Autodesk Inventor part; units mm, degrees
(part 2 of 2)
  arc A186 (143.0168, 108.2996) -> (148.9586, 106.0969) centre (168.8384, 168.8384) ccw
  arc A187 (149.6716, 82.58) -> (149.6716, 89.42) centre (146.2516, 86) ccw
  arc A188 (142.8316, 89.42) -> (142.8316, 82.58) centre (146.2516, 86) ccw
  arc A189 (129.9116, 82.58) -> (129.9116, 89.42) centre (126.4916, 86) ccw
  arc A190 (162.6162, 88.8364) -> (163.108, 82.58) centre (166.574, 86) ccw
  arc A191 (162.6162, 88.8364) -> (162.6167, 91.1656) centre (160.9905, 90.0014) ccw
  arc A192 (162.2055, 96.1467) -> (162.6167, 91.1656) centre (166.576, 94) ccw
  arc A193 (162.2055, 96.1467) -> (161.7567, 96.8671) centre (161.7567, 96.3671) ccw
  arc A194 (161.208, 75.1329) -> (163.108, 77.0329) centre (161.208, 77.0329) ccw
  arc A195 (149.6716, 77.0329) -> (151.5716, 75.1329) centre (151.5716, 77.0329) ccw
  line L125 (151.5716, 96.8671) -> (161.7567, 96.8671)
  line L126 (163.108, 82.58) -> (163.108, 77.0329)
  line L127 (161.208, 75.1329) -> (151.5716, 75.1329)
  line L128 (149.6716, 77.0329) -> (149.6716, 82.58)
  arc A196 (140.9316, 75.1329) -> (142.8316, 77.0329) centre (140.9316, 77.0329) ccw
  arc A197 (138.1595, 75.3626) -> (139.0651, 75.1329) centre (139.0651, 77.0329) ccw
  arc A198 (129.9116, 80.9656) -> (130.906, 79.2953) centre (131.8116, 80.9656) ccw
  arc A199 (130.906, 92.7047) -> (129.9116, 91.0344) centre (131.8116, 91.0344) ccw
  arc A200 (142.8316, 94.9671) -> (140.9316, 96.8671) centre (140.9316, 94.9671) ccw
  arc A201 (139.0651, 96.8671) -> (138.1595, 96.6374) centre (139.0651, 94.9671) ccw
  line L129 (130.906, 92.7047) -> (138.1595, 96.6374)
  line L130 (139.0651, 96.8671) -> (140.9316, 96.8671)
  line L131 (142.8316, 94.9671) -> (142.8316, 89.42)
  line L132 (142.8316, 82.58) -> (142.8316, 77.0329)
  line L133 (138.1595, 75.3626) -> (130.906, 79.2953)
  line L134 (129.9116, 80.9656) -> (129.9116, 82.58)
  line L135 (129.9116, 89.42) -> (129.9116, 91.0344)
  line L136 (139.0651, 75.1329) -> (140.9316, 75.1329)
  arc A202 (131.2701, 73.3555) -> (131.3324, 75.1447) centre (130.8558, 74.2656) ccw
  arc A203 (122.2131, 80.089) -> (118.7118, 78.848) centre (121.0215, 77.8913) ccw
  arc A204 (112.9272, 64.8827) -> (113.8511, 63.5) centre (113.8511, 64.5) ccw
  arc A205 (115.4267, 63.5) -> (116.072, 63.7361) centre (115.4267, 64.5) ccw
  arc A206 (131.2701, 73.3555) -> (116.072, 63.7361) centre (158.5315, 13.4685) ccw
  line L137 (115.4267, 63.5) -> (113.8511, 63.5)
  line L138 (112.9272, 64.8827) -> (118.7118, 78.848)
  line L139 (122.2131, 80.089) -> (131.3324, 75.1447)
  arc A207 (122.1239, 65.314) -> (122.7047, 63.5) centre (122.7047, 64.5) ccw
  arc A208 (148.9522, 65.9007) -> (150.6725, 68.8) centre (148.0207, 68.4135) ccw
  arc A209 (142.036, 63.5) -> (143.0168, 63.7004) centre (142.036, 66) ccw
  arc A210 (136.55, 72.3159) -> (134.8209, 72.401) centre (135.5967, 70.5576) ccw
  arc A211 (138.308, 71.3627) -> (139.7379, 71) centre (139.7379, 74) ccw
  line L140 (139.7379, 71) -> (146.5, 71)
  line L141 (146.5, 71) -> (146.5, 68.8)
  line L142 (146.5, 68.8) -> (150.6725, 68.8)
  line L143 (148.9522, 65.9007) -> (143.0168, 63.7004)
  line L144 (142.036, 63.5) -> (122.7047, 63.5)
  line L145 (138.308, 71.3627) -> (136.55, 72.3159)
  arc A212 (134.8209, 72.401) -> (122.1239, 65.314) centre (160.3459, 11.7536) ccw
  arc A213 (89.42, 29.1684) -> (82.58, 29.1684) centre (86, 25.7484) ccw
  arc A214 (82.58, 22.3284) -> (89.42, 22.3284) centre (86, 25.7484) ccw
  arc A215 (82.58, 42.0884) -> (89.42, 42.0884) centre (86, 45.5084) ccw
  arc A216 (75.1329, 10.792) -> (77.0329, 8.892) centre (77.0329, 10.792) ccw
  arc A217 (96.8671, 20.4284) -> (94.9671, 22.3284) centre (94.9671, 20.4284) ccw
  arc A218 (77.0329, 22.3284) -> (75.1329, 20.4284) centre (77.0329, 20.4284) ccw
  line L146 (77.0329, 22.3284) -> (82.58, 22.3284)
  line L147 (89.42, 22.3284) -> (94.9671, 22.3284)
  line L148 (75.1329, 20.4284) -> (75.1329, 10.792)
  line L149 (77.0329, 8.892) -> (82.58, 8.892)
  arc A219 (96.1467, 9.7945) -> (96.8671, 10.2433) centre (96.3671, 10.2433) ccw
  arc A220 (96.1467, 9.7945) -> (91.1656, 9.3833) centre (94, 5.424) ccw
  arc A221 (88.8364, 9.3838) -> (91.1656, 9.3833) centre (90.0014, 11.0095) ccw
  arc A222 (88.8364, 9.3838) -> (82.58, 8.892) centre (86, 5.426) ccw
  line L150 (96.8671, 10.2433) -> (96.8671, 20.4284)
  arc A223 (94.9671, 29.1684) -> (96.8671, 31.0684) centre (94.9671, 31.0684) ccw
  arc A224 (96.8671, 32.9349) -> (96.6374, 33.8405) centre (94.9671, 32.9349) ccw
  arc A225 (75.1329, 31.0684) -> (77.0329, 29.1684) centre (77.0329, 31.0684) ccw
  arc A226 (75.3626, 33.8405) -> (75.1329, 32.9349) centre (77.0329, 32.9349) ccw
  arc A227 (80.9656, 42.0884) -> (79.2953, 41.094) centre (80.9656, 40.1884) ccw
  arc A228 (92.7047, 41.094) -> (91.0344, 42.0884) centre (91.0344, 40.1884) ccw
  line L151 (96.8671, 32.9349) -> (96.8671, 31.0684)
  line L152 (94.9671, 29.1684) -> (89.42, 29.1684)
  line L153 (96.6374, 33.8405) -> (92.7047, 41.094)
  line L154 (91.0344, 42.0884) -> (89.42, 42.0884)
  line L155 (82.58, 42.0884) -> (80.9656, 42.0884)
  line L156 (79.2953, 41.094) -> (75.3626, 33.8405)
  line L157 (75.1329, 32.9349) -> (75.1329, 31.0684)
  line L158 (77.0329, 29.1684) -> (82.58, 29.1684)
  arc A229 (119.0041, 59.6222) -> (118.6767, 60.5) centre (118.6767, 60) ccw
  arc A230 (114, 60.5) -> (111.5, 58) centre (114, 58) ccw
  arc A231 (111.5, 53.3233) -> (112.3778, 52.9958) centre (112, 53.3233) ccw
  line L159 (114, 60.5) -> (118.6767, 60.5)
  line L160 (111.5, 58) -> (111.5, 53.3233)
  arc A232 (119.0041, 59.6222) -> (112.3778, 52.9958) centre (162.1005, 9.8995) ccw
  arc A233 (123.9045, 60.5) -> (122.6628, 60.0679) centre (123.9045, 58.5) ccw
  arc A234 (111.9321, 49.3372) -> (111.5, 48.0955) centre (113.5, 48.0955) ccw
  arc A235 (133.455, 58.6568) -> (132.9173, 60.5) centre (132.9173, 59.5) ccw
  arc A236 (111.5, 39.0827) -> (113.3432, 38.545) centre (112.5, 39.0827) ccw
  line L161 (111.5, 39.0827) -> (111.5, 48.0955)
  arc A237 (122.6628, 60.0679) -> (111.9321, 49.3372) centre (163.5147, 8.4853) ccw
  arc A238 (133.455, 58.6568) -> (113.3432, 38.545) centre (168.8384, 3.1616) ccw
  line L162 (132.9173, 60.5) -> (123.9045, 60.5)
  arc A239 (93.152, 53.2882) -> (91.911, 49.7869) centre (94.1087, 50.9785) ccw
  arc A240 (108.5, 58.1489) -> (107.1173, 59.0728) centre (107.5, 58.1489) ccw
  arc A241 (108.2639, 55.928) -> (108.5, 56.5733) centre (107.5, 56.5733) ccw
  arc A242 (96.8553, 40.6676) -> (98.6445, 40.7299) centre (97.7344, 41.1442) ccw
  arc A243 (108.2639, 55.928) -> (98.6445, 40.7299) centre (158.5315, 13.4685) ccw
  line L163 (108.5, 56.5733) -> (108.5, 58.1489)
  line L164 (107.1173, 59.0728) -> (93.152, 53.2882)
  line L165 (91.911, 49.7869) -> (96.8553, 40.6676)
  arc A244 (101, 32.2621) -> (100.6373, 33.692) centre (98, 32.2621) ccw
  arc A245 (99.599, 37.1791) -> (99.6841, 35.45) centre (101.4423, 36.4033) ccw
  arc A246 (108.2996, 28.9832) -> (108.5, 29.964) centre (106, 29.964) ccw
  arc A247 (103.2, 21.3275) -> (106.0968, 23.0414) centre (103.5865, 23.9793) ccw
  arc A248 (108.5, 49.2953) -> (106.686, 49.8761) centre (107.5, 49.2953) ccw
  arc A249 (106.686, 49.8761) -> (99.599, 37.1791) centre (160.2464, 11.6541) ccw
  line L166 (108.5, 49.2953) -> (108.5, 29.964)
  line L167 (100.6373, 33.692) -> (99.6841, 35.45)
  arc A250 (108.2996, 28.9832) -> (106.0968, 23.0414) centre (168.8384, 3.1616) ccw
  line L168 (103.2, 21.3275) -> (103.2, 25.5)
  line L169 (103.2, 25.5) -> (101, 25.5)
  line L170 (101, 25.5) -> (101, 32.2621)
  arc A251 (65.9031, 23.0414) -> (68.8, 21.3275) centre (68.4135, 23.9793) ccw
  arc A252 (63.5, 29.964) -> (63.7004, 28.9832) centre (66, 29.964) ccw
  arc A253 (71.3627, 33.692) -> (71, 32.2621) centre (74, 32.2621) ccw
  arc A254 (72.3159, 35.45) -> (72.401, 37.1791) centre (70.5576, 36.4033) ccw
  arc A255 (65.314, 49.8761) -> (63.5, 49.2953) centre (64.5, 49.2953) ccw
  arc A256 (65.9031, 23.0414) -> (63.7004, 28.9832) centre (3.1615, 3.1616) ccw
  arc A257 (72.401, 37.1791) -> (65.314, 49.8761) centre (11.7536, 11.6541) ccw
  line L171 (68.8, 21.3275) -> (68.8, 25.5)
  line L172 (68.8, 25.5) -> (71, 25.5)
  line L173 (71, 25.5) -> (71, 32.2621)
  line L174 (71.3627, 33.692) -> (72.3159, 35.45)
  line L175 (63.5, 29.964) -> (63.5, 49.2953)
  arc A258 (80.089, 49.7869) -> (78.848, 53.2882) centre (77.8913, 50.9785) ccw
  arc A259 (64.8827, 59.0728) -> (63.5, 58.1489) centre (64.5, 58.1489) ccw
  arc A260 (63.5, 56.5733) -> (63.7361, 55.928) centre (64.5, 56.5733) ccw
  arc A261 (73.3555, 40.7299) -> (75.1447, 40.6676) centre (74.2656, 41.1442) ccw
  line L176 (75.1447, 40.6676) -> (80.089, 49.7869)
  line L177 (78.848, 53.2882) -> (64.8827, 59.0728)
  line L178 (63.5, 58.1489) -> (63.5, 56.5733)
  arc A262 (73.3555, 40.7299) -> (63.7361, 55.928) centre (13.4685, 13.4685) ccw
  arc A263 (151.5716, 96.8671) -> (149.6716, 94.9671) centre (151.5716, 94.9671) ccw
  line L179 (149.6716, 94.9671) -> (149.6716, 89.42)
  arc A264 (91.911, 122.2131) -> (93.152, 118.7118) centre (94.1087, 121.0215) ccw
  line L180 (93.152, 118.7118) -> (107.1173, 112.9272)
  arc A265 (75.8533, 162.2055) -> (80.8344, 162.6167) centre (78, 166.576) ccw
  arc A266 (75.8533, 162.2055) -> (75.1329, 161.7567) centre (75.6329, 161.7567) ccw
  line L181 (75.1329, 161.7567) -> (75.1329, 151.5716)
  arc A267 (75.1329, 139.0651) -> (75.3626, 138.1595) centre (77.0329, 139.0651) ccw
  line L182 (75.1329, 139.0651) -> (75.1329, 140.9316)
  line L183 (75.3626, 138.1595) -> (79.2953, 130.906)
  arc A268 (63.6264, 105.803) -> (61.8724, 104.5705) centre (63.7201, 103.8052) ccw
  arc A269 (67.4295, 110.1276) -> (66.197, 108.3735) centre (68.1948, 108.2799) ccw
  arc A270 (63.6264, 105.803) -> (66.197, 108.3735) centre (63.5, 108.5) ccw
  arc A271 (61.8724, 67.4295) -> (63.6264, 66.197) centre (63.7201, 68.1948) ccw
  arc A272 (66.197, 63.6265) -> (67.4295, 61.8724) centre (68.1948, 63.7201) ccw
  arc A273 (66.197, 63.6265) -> (63.6264, 66.197) centre (63.5, 63.5) ccw
  line L184 (67.4295, 61.8724) -> (82.0705, 55.8078)
  line L185 (61.8724, 67.4295) -> (55.8078, 82.0705)
  line L186 (55.8078, 89.9295) -> (61.8724, 104.5705)
  line L187 (67.4295, 110.1276) -> (82.0705, 116.1922)
  arc A274 (82.0705, 55.8078) -> (84.1823, 56.1767) centre (82.8359, 57.6556) ccw
  arc A275 (87.8177, 56.1767) -> (89.9295, 55.8078) centre (89.1641, 57.6556) ccw
  arc A276 (87.8177, 56.1767) -> (84.1823, 56.1767) centre (86, 54.1802) ccw
  line L188 (89.9295, 55.8078) -> (104.5705, 61.8724)
  arc A277 (31.0684, 96.8671) -> (29.1684, 94.9671) centre (31.0684, 94.9671) ccw
  line L189 (31.0684, 96.8671) -> (32.9349, 96.8671)
  line L190 (29.1684, 89.42) -> (29.1684, 94.9671)
  circle A278 centre (54.1802, 86) radius 1.6
  circle A279 centre (63.5, 108.5) radius 1.6
  circle A280 centre (86, 117.8198) radius 1.6
  circle A281 centre (108.5, 108.5) radius 1.6
  circle A282 centre (117.8198, 86) radius 1.6
  circle A283 centre (108.5, 63.5) radius 1.6
  circle A284 centre (63.5, 63.5) radius 1.6
  circle A285 centre (86, 54.1802) radius 1.6
  arc A286 (56.1767, 84.1823) -> (56.1767, 87.8177) centre (54.1802, 86) ccw
  arc A287 (55.8078, 89.9295) -> (56.1767, 87.8177) centre (57.6556, 89.1641) ccw
  arc A288 (56.1767, 84.1823) -> (55.8078, 82.0705) centre (57.6556, 82.8359) ccw
  arc A289 (63.6264, 105.803) -> (66.197, 108.3735) centre (63.5, 108.5) ccw
  arc A290 (63.6264, 105.803) -> (61.8724, 104.5705) centre (63.7201, 103.8052) ccw
  arc A291 (67.4295, 110.1276) -> (66.197, 108.3735) centre (68.1948, 108.2799) ccw
  arc A292 (84.1823, 115.8233) -> (87.8177, 115.8233) centre (86, 117.8198) ccw
  arc A293 (89.9295, 116.1922) -> (87.8177, 115.8233) centre (89.1641, 114.3444) ccw
  arc A294 (84.1823, 115.8233) -> (82.0705, 116.1922) centre (82.8359, 114.3444) ccw
  arc A295 (105.803, 108.3735) -> (108.3735, 105.803) centre (108.5, 108.5) ccw
  arc A296 (110.1276, 104.5705) -> (108.3735, 105.803) centre (108.2799, 103.8052) ccw
  arc A297 (105.803, 108.3735) -> (104.5705, 110.1276) centre (103.8052, 108.2799) ccw
  arc A298 (115.8233, 87.8177) -> (115.8233, 84.1823) centre (117.8198, 86) ccw
  arc A299 (116.1922, 82.0705) -> (115.8233, 84.1823) centre (114.3444, 82.8359) ccw
  arc A300 (115.8233, 87.8177) -> (116.1922, 89.9295) centre (114.3444, 89.1641) ccw
  arc A301 (66.197, 63.6265) -> (63.6264, 66.197) centre (63.5, 63.5) ccw
  arc A302 (61.8724, 67.4295) -> (63.6264, 66.197) centre (63.7201, 68.1948) ccw
  arc A303 (66.197, 63.6265) -> (67.4295, 61.8724) centre (68.1948, 63.7201) ccw
  arc A304 (87.8177, 56.1767) -> (84.1823, 56.1767) centre (86, 54.1802) ccw
  arc A305 (82.0705, 55.8078) -> (84.1823, 56.1767) centre (82.8359, 57.6556) ccw
  arc A306 (87.8177, 56.1767) -> (89.9295, 55.8078) centre (89.1641, 57.6556) ccw
  arc A307 (108.3735, 66.197) -> (105.803, 63.6265) centre (108.5, 63.5) ccw
  arc A308 (104.5705, 61.8724) -> (105.803, 63.6265) centre (103.8052, 63.7201) ccw
  arc A309 (108.3735, 66.197) -> (110.1276, 67.4295) centre (108.2799, 68.1948) ccw
  line L191 (55.8078, 82.0705) -> (61.8724, 67.4295)
  line L192 (67.4295, 61.8724) -> (82.0705, 55.8078)
  line L193 (89.9295, 55.8078) -> (104.5705, 61.8724)
  line L194 (110.1276, 67.4295) -> (116.1922, 82.0705)
  line L195 (116.1922, 89.9295) -> (110.1276, 104.5705)
  line L196 (104.5705, 110.1276) -> (89.9295, 116.1922)
  line L197 (82.0705, 116.1922) -> (67.4295, 110.1276)
  line L198 (61.8724, 104.5705) -> (55.8078, 89.9295)
  line L199 (0, 99.484) -> (0, 101)
  arc A310 (0, 99.484) -> (0.217, 98.5779) centre (2, 99.484) ccw
  line L200 (0, 101) -> (6.5, 101)
  line L201 (6.5, 101) -> (6.5, 103.2)
  line L202 (6.5, 103.2) -> (0, 103.2)
  line L203 (0, 103.2) -> (0, 106.2)
  line L204 (71, 172) -> (71, 165.5)
  line L205 (71, 165.5) -> (68.8, 165.5)
  line L206 (68.8, 165.5) -> (68.8, 172)
  line L207 (68.8, 172) -> (65.8, 172)
  arc A311 (0, 106.2) -> (65.8, 172) centre (0, 172) ccw
  line L208 (101, 172) -> (101, 165.5)
  line L209 (101, 165.5) -> (103.2, 165.5)
  line L210 (103.2, 165.5) -> (103.2, 172)
  line L211 (103.2, 172) -> (106.2, 172)
  line L212 (172, 101) -> (165.5, 101)
  line L213 (165.5, 101) -> (165.5, 103.2)
  line L214 (165.5, 103.2) -> (172, 103.2)
  line L215 (172, 103.2) -> (172, 106.2)
  arc A312 (106.2, 172) -> (172, 106.2) centre (172, 172) ccw
  line L216 (0, 71) -> (6.5, 71)
  line L217 (6.5, 71) -> (6.5, 68.8)
  line L218 (6.5, 68.8) -> (0, 68.8)
  line L219 (0, 68.8) -> (0, 65.8)
  line L220 (71, 0) -> (71, 6.5)
  line L221 (71, 6.5) -> (68.8, 6.5)
  line L222 (68.8, 6.5) -> (68.8, 0)
  line L223 (68.8, 0) -> (65.8, 0)
  arc A313 (65.8, 0) -> (0, 65.8) centre (0, 0) ccw
  line L224 (101, 0) -> (101, 6.5)
  line L225 (101, 6.5) -> (103.2, 6.5)
  line L226 (103.2, 6.5) -> (103.2, 0)
  line L227 (103.2, 0) -> (106.2, 0)
  line L228 (172, 71) -> (165.5, 71)
  line L229 (165.5, 71) -> (165.5, 68.8)
  line L230 (165.5, 68.8) -> (172, 68.8)
  line L231 (172, 68.8) -> (172, 65.8)
  arc A314 (172, 65.8) -> (106.2, 0) centre (172, 0) ccw
  circle A315 centre (45.5084, 86) radius 2.1
  circle A316 centre (5.472, 86) radius 1.6
  circle A317 centre (25.7484, 86) radius 1.6
  line L232 (10.792, 96.8671) -> (20.4284, 96.8671)
  arc A318 (10.792, 96.8671) -> (8.892, 94.9671) centre (10.792, 94.9671) ccw
  line L233 (8.892, 94.9671) -> (8.892, 89.42)
  line L234 (22.3284, 89.42) -> (22.3284, 94.9671)
  arc A319 (22.3284, 94.9671) -> (20.4284, 96.8671) centre (20.4284, 94.9671) ccw
  line L235 (10.2433, 75.1329) -> (20.4284, 75.1329)
  line L236 (22.3284, 82.58) -> (22.3284, 77.0329)
  arc A320 (20.4284, 75.1329) -> (22.3284, 77.0329) centre (20.4284, 77.0329) ccw
  arc A321 (9.3838, 83.1636) -> (8.892, 89.42) centre (5.426, 86) ccw
  arc A322 (22.3284, 89.42) -> (22.3284, 82.58) centre (25.7484, 86) ccw
  line L237 (32.9349, 96.8671) -> (31.0684, 96.8671)
  line L238 (29.1684, 89.42) -> (29.1684, 94.9671)
  arc A323 (31.0684, 96.8671) -> (29.1684, 94.9671) centre (31.0684, 94.9671) ccw
  arc A324 (29.1684, 82.58) -> (29.1684, 89.42) centre (25.7484, 86) ccw
  line L239 (33.8405, 96.6374) -> (41.094, 92.7047)
  arc A325 (33.8405, 96.6374) -> (32.9349, 96.8671) centre (32.9349, 94.9671) ccw
  line L240 (42.0884, 91.0344) -> (42.0884, 89.42)
  arc A326 (42.0884, 91.0344) -> (41.094, 92.7047) centre (40.1884, 91.0344) ccw
  arc A327 (42.0884, 89.42) -> (42.0884, 82.58) centre (45.5084, 86) ccw
  line L241 (32.9349, 75.1329) -> (31.0684, 75.1329)
  line L242 (29.1684, 82.58) -> (29.1684, 77.0329)
  arc A328 (29.1684, 77.0329) -> (31.0684, 75.1329) centre (31.0684, 77.0329) ccw
  line L243 (33.8405, 75.3626) -> (41.094, 79.2953)
  arc A329 (32.9349, 75.1329) -> (33.8405, 75.3626) centre (32.9349, 77.0329) ccw
  line L244 (42.0884, 80.9656) -> (42.0884, 82.58)
  arc A330 (41.094, 79.2953) -> (42.0884, 80.9656) centre (40.1884, 80.9656) ccw
  circle A331 centre (126.4916, 86) radius 2.1
  circle A332 centre (146.2516, 86) radius 1.6
  line L245 (161.7567, 96.8671) -> (151.5716, 96.8671)
  line L246 (149.6716, 89.42) -> (149.6716, 94.9671)
  arc A333 (151.5716, 96.8671) -> (149.6716, 94.9671) centre (151.5716, 94.9671) ccw
  line L247 (161.208, 75.1329) -> (151.5716, 75.1329)
  line L248 (149.6716, 82.58) -> (149.6716, 77.0329)
  arc A334 (149.6716, 77.0329) -> (151.5716, 75.1329) centre (151.5716, 77.0329) ccw
  arc A335 (149.6716, 82.58) -> (149.6716, 89.42) centre (146.2516, 86) ccw
  line L249 (139.0651, 96.8671) -> (140.9316, 96.8671)
  line L250 (142.8316, 89.42) -> (142.8316, 94.9671)
  arc A336 (142.8316, 94.9671) -> (140.9316, 96.8671) centre (140.9316, 94.9671) ccw
  arc A337 (142.8316, 89.42) -> (142.8316, 82.58) centre (146.2516, 86) ccw
  line L251 (138.1595, 96.6374) -> (130.906, 92.7047)
  arc A338 (139.0651, 96.8671) -> (138.1595, 96.6374) centre (139.0651, 94.9671) ccw
  line L252 (129.9116, 91.0344) -> (129.9116, 89.42)
  arc A339 (130.906, 92.7047) -> (129.9116, 91.0344) centre (131.8116, 91.0344) ccw
  arc A340 (129.9116, 82.58) -> (129.9116, 89.42) centre (126.4916, 86) ccw
  line L253 (139.0651, 75.1329) -> (140.9316, 75.1329)
  line L254 (142.8316, 82.58) -> (142.8316, 77.0329)
  arc A341 (140.9316, 75.1329) -> (142.8316, 77.0329) centre (140.9316, 77.0329) ccw
  line L255 (138.1595, 75.3626) -> (130.906, 79.2953)
  arc A342 (138.1595, 75.3626) -> (139.0651, 75.1329) centre (139.0651, 77.0329) ccw
  line L256 (129.9116, 80.9656) -> (129.9116, 82.58)
  arc A343 (129.9116, 80.9656) -> (130.906, 79.2953) centre (131.8116, 80.9656) ccw
  circle A344 centre (86, 126.4916) radius 2.1
  circle A345 centre (86, 146.2516) radius 1.6
  line L257 (75.1329, 161.7567) -> (75.1329, 151.5716)
  line L258 (82.58, 149.6716) -> (77.0329, 149.6716)
  arc A346 (75.1329, 151.5716) -> (77.0329, 149.6716) centre (77.0329, 151.5716) ccw
  line L259 (96.8671, 161.208) -> (96.8671, 151.5716)
  line L260 (89.42, 149.6716) -> (94.9671, 149.6716)
  arc A347 (94.9671, 149.6716) -> (96.8671, 151.5716) centre (94.9671, 151.5716) ccw
  arc A348 (89.42, 149.6716) -> (82.58, 149.6716) centre (86, 146.2516) ccw
  line L261 (75.1329, 139.0651) -> (75.1329, 140.9316)
  line L262 (82.58, 142.8316) -> (77.0329, 142.8316)
  arc A349 (77.0329, 142.8316) -> (75.1329, 140.9316) centre (77.0329, 140.9316) ccw
  arc A350 (82.58, 142.8316) -> (89.42, 142.8316) centre (86, 146.2516) ccw
  line L263 (75.3626, 138.1595) -> (79.2953, 130.906)
  arc A351 (75.1329, 139.0651) -> (75.3626, 138.1595) centre (77.0329, 139.0651) ccw
  arc A352 (96.8671, 20.4284) -> (94.9671, 22.3284) centre (94.9671, 20.4284) ccw
  line L264 (80.9656, 129.9116) -> (82.58, 129.9116)
  arc A353 (79.2953, 130.906) -> (80.9656, 129.9116) centre (80.9656, 131.8116) ccw
  arc A354 (89.42, 129.9116) -> (82.58, 129.9116) centre (86, 126.4916) ccw
  line L265 (96.8671, 139.0651) -> (96.8671, 140.9316)
  line L266 (89.42, 142.8316) -> (94.9671, 142.8316)
  arc A355 (96.8671, 140.9316) -> (94.9671, 142.8316) centre (94.9671, 140.9316) ccw
  line L267 (96.6374, 138.1595) -> (92.7047, 130.906)
  line L268 (96.8671, 32.9349) -> (96.8671, 31.0684)
  arc A356 (96.6374, 138.1595) -> (96.8671, 139.0651) centre (94.9671, 139.0651) ccw
  line L269 (91.0344, 129.9116) -> (89.42, 129.9116)
  arc A357 (91.0344, 129.9116) -> (92.7047, 130.906) centre (91.0344, 131.8116) ccw
  circle A358 centre (86, 45.5084) radius 2.1
  circle A359 centre (86, 25.7484) radius 1.6
  line L270 (96.8671, 10.2433) -> (96.8671, 20.4284)
  line L271 (89.42, 22.3284) -> (94.9671, 22.3284)
  line L272 (75.1329, 10.792) -> (75.1329, 20.4284)
  arc A360 (92.7047, 41.094) -> (91.0344, 42.0884) centre (91.0344, 40.1884) ccw
  line L273 (82.58, 22.3284) -> (77.0329, 22.3284)
  line L274 (82.58, 29.1684) -> (77.0329, 29.1684)
  arc A361 (77.0329, 22.3284) -> (75.1329, 20.4284) centre (77.0329, 20.4284) ccw
  arc A362 (82.58, 22.3284) -> (89.42, 22.3284) centre (86, 25.7484) ccw
  line L275 (80.9656, 42.0884) -> (82.58, 42.0884)
  line L276 (89.42, 29.1684) -> (94.9671, 29.1684)
  arc A363 (94.9671, 29.1684) -> (96.8671, 31.0684) centre (94.9671, 31.0684) ccw
  arc A364 (89.42, 29.1684) -> (82.58, 29.1684) centre (86, 25.7484) ccw
  line L277 (96.6374, 33.8405) -> (92.7047, 41.094)
  arc A365 (96.8671, 32.9349) -> (96.6374, 33.8405) centre (94.9671, 32.9349) ccw
  line L278 (91.0344, 42.0884) -> (89.42, 42.0884)
  arc A366 (82.58, 42.0884) -> (89.42, 42.0884) centre (86, 45.5084) ccw
  line L279 (75.1329, 32.9349) -> (75.1329, 31.0684)
  arc A367 (75.1329, 31.0684) -> (77.0329, 29.1684) centre (77.0329, 31.0684) ccw
  arc A368 (80.9656, 42.0884) -> (79.2953, 41.094) centre (80.9656, 40.1884) ccw
  line L280 (75.3626, 33.8405) -> (79.2953, 41.094)
  arc A369 (75.3626, 33.8405) -> (75.1329, 32.9349) centre (77.0329, 32.9349) ccw
  line L281 (2.052, 94.4881) -> (2.052, 89.42)
  arc A370 (2.052, 89.42) -> (1.5587, 83.1656) centre (5.518, 86) ccw
  line L282 (0.217, 98.5779) -> (1.835, 95.3941)
  arc A371 (2.052, 94.4881) -> (1.835, 95.3941) centre (0.052, 94.4881) ccw
  arc A372 (0.217, 73.4221) -> (0, 72.516) centre (2, 72.516) ccw
  line L283 (0.217, 73.4221) -> (0.8629, 74.6931)
  line L284 (0, 71) -> (0, 72.516)
  circle A373 centre (5.47, 78) radius 1.6
  arc A374 (9.7945, 75.8533) -> (9.3832, 80.8344) centre (5.424, 78) ccw
  arc A375 (9.7945, 75.8533) -> (10.2433, 75.1329) centre (10.2433, 75.6329) ccw
  arc A376 (9.3838, 83.1636) -> (9.3832, 80.8344) centre (11.0095, 81.9986) ccw
  arc A377 (1.5581, 80.8364) -> (0.9538, 76.2982) centre (5.516, 78) ccw
  arc A378 (1.5581, 80.8364) -> (1.5587, 83.1656) centre (-0.0675, 82.0014) ccw
  arc A379 (0.8629, 74.6931) -> (0.9538, 76.2982) centre (-0.9201, 75.5992) ccw
  line L285 (172, 72.516) -> (172, 71)
  arc A380 (172, 72.516) -> (171.783, 73.4221) centre (170, 72.516) ccw
  circle A381 centre (166.528, 86) radius 1.6
  arc A382 (161.208, 75.1329) -> (163.108, 77.0329) centre (161.208, 77.0329) ccw
  line L286 (163.108, 77.0329) -> (163.108, 82.58)
  arc A383 (162.6162, 88.8364) -> (163.108, 82.58) centre (166.574, 86) ccw
  line L287 (169.948, 77.5119) -> (169.948, 82.58)
  arc A384 (169.948, 82.58) -> (170.4413, 88.8344) centre (166.482, 86) ccw
  line L288 (171.783, 73.4221) -> (170.165, 76.6059)
  arc A385 (169.948, 77.5119) -> (170.165, 76.6059) centre (171.948, 77.5119) ccw
  arc A386 (171.783, 98.5779) -> (172, 99.484) centre (170, 99.484) ccw
  line L289 (171.783, 98.5779) -> (171.1371, 97.3069)
  line L290 (172, 101) -> (172, 99.484)
  circle A387 centre (166.53, 94) radius 1.6
  arc A388 (162.2055, 96.1467) -> (162.6167, 91.1656) centre (166.576, 94) ccw
  arc A389 (162.2055, 96.1467) -> (161.7567, 96.8671) centre (161.7567, 96.3671) ccw
  arc A390 (162.6162, 88.8364) -> (162.6167, 91.1656) centre (160.9905, 90.0014) ccw
  arc A391 (170.4419, 91.1636) -> (171.0462, 95.7018) centre (166.484, 94) ccw
  arc A392 (170.4419, 91.1636) -> (170.4413, 88.8344) centre (172.0675, 89.9986) ccw
  arc A393 (171.1371, 97.3069) -> (171.0462, 95.7018) centre (172.92, 96.4008) ccw
  line L291 (72.516, 0) -> (71, 0)
  arc A394 (72.516, 0) -> (73.4221, 0.217) centre (72.516, 2) ccw
  circle A395 centre (86, 5.472) radius 1.6
  arc A396 (75.1329, 10.792) -> (77.0329, 8.892) centre (77.0329, 10.792) ccw
  line L292 (77.0329, 8.892) -> (82.58, 8.892)
  arc A397 (88.8364, 9.3838) -> (82.58, 8.892) centre (86, 5.426) ccw
  line L293 (77.5119, 2.052) -> (82.58, 2.052)
  arc A398 (82.58, 2.052) -> (88.8344, 1.5587) centre (86, 5.518) ccw
  line L294 (73.4221, 0.217) -> (76.6059, 1.835)
  arc A399 (77.5119, 2.052) -> (76.6059, 1.835) centre (77.5119, 0.052) ccw
  arc A400 (98.5779, 0.217) -> (99.484, 0) centre (99.484, 2) ccw
  line L295 (98.5779, 0.217) -> (97.3069, 0.8629)
  line L296 (101, 0) -> (99.484, 0)
  circle A401 centre (94, 5.47) radius 1.6
  arc A402 (96.1467, 9.7945) -> (91.1656, 9.3833) centre (94, 5.424) ccw
  arc A403 (96.1467, 9.7945) -> (96.8671, 10.2433) centre (96.3671, 10.2433) ccw
  arc A404 (88.8364, 9.3838) -> (91.1656, 9.3833) centre (90.0014, 11.0095) ccw
  arc A405 (91.1636, 1.5581) -> (95.7018, 0.9538) centre (94, 5.516) ccw
  arc A406 (91.1636, 1.5581) -> (88.8344, 1.5587) centre (89.9986, -0.0675) ccw
  arc A407 (97.3069, 0.8629) -> (95.7018, 0.9538) centre (96.4008, -0.92) ccw
  line L297 (99.484, 172) -> (101, 172)
  arc A408 (99.484, 172) -> (98.5779, 171.783) centre (99.484, 170) ccw
  circle A409 centre (86, 166.528) radius 1.6
  arc A410 (96.8671, 161.208) -> (94.9671, 163.108) centre (94.9671, 161.208) ccw
  line L298 (94.9671, 163.108) -> (89.42, 163.108)
  arc A411 (83.1636, 162.6162) -> (89.42, 163.108) centre (86, 166.574) ccw
  line L299 (94.4881, 169.948) -> (89.42, 169.948)
  arc A412 (89.42, 169.948) -> (83.1656, 170.4413) centre (86, 166.482) ccw
  line L300 (98.5779, 171.783) -> (95.3941, 170.165)
  arc A413 (94.4881, 169.948) -> (95.3941, 170.165) centre (94.4881, 171.948) ccw
  arc A414 (73.4221, 171.783) -> (72.516, 172) centre (72.516, 170) ccw
  line L301 (73.4221, 171.783) -> (74.6931, 171.1371)
  line L302 (71, 172) -> (72.516, 172)
  circle A415 centre (78, 166.53) radius 1.6
  arc A416 (75.8533, 162.2055) -> (80.8344, 162.6167) centre (78, 166.576) ccw
  arc A417 (75.8533, 162.2055) -> (75.1329, 161.7567) centre (75.6329, 161.7567) ccw
  arc A418 (83.1636, 162.6162) -> (80.8344, 162.6167) centre (81.9986, 160.9905) ccw
  arc A419 (80.8364, 170.4419) -> (76.2982, 171.0462) centre (78, 166.484) ccw
  arc A420 (80.8364, 170.4419) -> (83.1656, 170.4413) centre (82.0014, 172.0675) ccw
  arc A421 (74.6931, 171.1371) -> (76.2982, 171.0462) centre (75.5992, 172.92) ccw
  arc A422 (38.545, 113.3432) -> (58.6568, 133.455) centre (3.1615, 168.8384) ccw
  arc A423 (38.545, 113.3432) -> (39.0827, 111.5) centre (39.0827, 112.5) ccw
  arc A424 (60.5, 132.9173) -> (58.6568, 133.455) centre (59.5, 132.9173) ccw
  line L303 (58, 111.5) -> (53.3233, 111.5)
  line L304 (48.0955, 111.5) -> (39.0827, 111.5)
  line L305 (60.5, 114) -> (60.5, 118.6767)
  line L306 (60.5, 123.9045) -> (60.5, 132.9173)
  arc A425 (58, 111.5) -> (60.5, 114) centre (58, 114) ccw
  circle A426 centre (53.1485, 53.0665) radius 3.15
  circle A427 centre (48.4963, 57.6887) radius 1.6
  circle A428 centre (57.6887, 48.4963) radius 1.6
  line L307 (63.5, 122.7047) -> (63.5, 142.036)
  arc A429 (63.7361, 116.072) -> (73.3555, 131.2701) centre (13.4685, 158.5315) ccw
  arc A430 (63.7361, 116.072) -> (63.5, 115.4267) centre (64.5, 115.4267) ccw
  arc A431 (75.1447, 131.3324) -> (73.3555, 131.2701) centre (74.2656, 130.8558) ccw
  arc A432 (63.7004, 143.0168) -> (65.9031, 148.9586) centre (3.1615, 168.8384) ccw
  arc A433 (63.7004, 143.0168) -> (63.5, 142.036) centre (66, 142.036) ccw
  arc A434 (68.8, 150.6725) -> (65.9031, 148.9586) centre (68.4135, 148.0207) ccw
  line L308 (71.3627, 138.308) -> (72.3159, 136.55)
  line L309 (71, 146.5) -> (71, 139.7379)
  arc A435 (71, 139.7379) -> (71.3627, 138.308) centre (74, 139.7379) ccw
  arc A436 (49.3372, 111.9321) -> (60.0679, 122.6628) centre (8.4853, 163.5147) ccw
  arc A437 (48.0955, 111.5) -> (49.3372, 111.9321) centre (48.0955, 113.5) ccw
  arc A438 (60.0679, 122.6628) -> (60.5, 123.9045) centre (58.5, 123.9045) ccw
  arc A439 (52.9958, 112.3778) -> (59.6222, 119.0042) centre (9.8995, 162.1005) ccw
  arc A440 (52.9958, 112.3778) -> (53.3233, 111.5) centre (53.3233, 112) ccw
  arc A441 (60.5, 118.6767) -> (59.6222, 119.0042) centre (60, 118.6767) ccw
  arc A442 (113.3432, 133.455) -> (133.455, 113.3432) centre (168.8384, 168.8384) ccw
  arc A443 (132.9173, 111.5) -> (133.455, 113.3432) centre (132.9173, 112.5) ccw
  arc A444 (113.3432, 133.455) -> (111.5, 132.9173) centre (112.5, 132.9173) ccw
  line L310 (114, 111.5) -> (118.6767, 111.5)
  line L311 (123.9045, 111.5) -> (132.9173, 111.5)
  line L312 (111.5, 114) -> (111.5, 118.6767)
  line L313 (111.5, 123.9045) -> (111.5, 132.9173)
  arc A445 (111.5, 114) -> (114, 111.5) centre (114, 114) ccw
  arc A446 (111.9321, 122.6628) -> (122.6628, 111.9321) centre (163.5147, 163.5147) ccw
  arc A447 (122.6628, 111.9321) -> (123.9045, 111.5) centre (123.9045, 113.5) ccw
  arc A448 (111.5, 123.9045) -> (111.9321, 122.6628) centre (113.5, 123.9045) ccw
  arc A449 (112.3778, 119.0042) -> (119.0041, 112.3778) centre (162.1005, 162.1005) ccw
  arc A450 (118.6767, 111.5) -> (119.0041, 112.3778) centre (118.6767, 112) ccw
  arc A451 (112.3778, 119.0042) -> (111.5, 118.6767) centre (112, 118.6767) ccw
  arc A452 (133.455, 58.6568) -> (113.3432, 38.545) centre (168.8384, 3.1616) ccw
  arc A453 (133.455, 58.6568) -> (132.9173, 60.5) centre (132.9173, 59.5) ccw
  arc A454 (111.5, 39.0827) -> (113.3432, 38.545) centre (112.5, 39.0827) ccw
  line L314 (114, 60.5) -> (118.6767, 60.5)
  line L315 (123.9045, 60.5) -> (132.9173, 60.5)
  line L316 (111.5, 58) -> (111.5, 53.3233)
  line L317 (111.5, 48.0955) -> (111.5, 39.0827)
  arc A455 (114, 60.5) -> (111.5, 58) centre (114, 58) ccw
  arc A456 (122.6628, 60.0679) -> (111.9321, 49.3372) centre (163.5147, 8.4853) ccw
  arc A457 (123.9045, 60.5) -> (122.6628, 60.0679) centre (123.9045, 58.5) ccw
  arc A458 (111.9321, 49.3372) -> (111.5, 48.0955) centre (113.5, 48.0955) ccw
  arc A459 (119.0041, 59.6222) -> (112.3778, 52.9958) centre (162.1005, 9.8995) ccw
  arc A460 (119.0041, 59.6222) -> (118.6767, 60.5) centre (118.6767, 60) ccw
  arc A461 (111.5, 53.3233) -> (112.3778, 52.9958) centre (112, 53.3233) ccw
  line L318 (58, 60.5) -> (53.3233, 60.5)
  line L319 (60.5, 58) -> (60.5, 53.3233)
  arc A462 (60.5, 58) -> (58, 60.5) centre (58, 58) ccw
  arc A463 (59.6222, 52.9958) -> (52.9958, 59.6222) centre (9.8995, 9.8995) ccw
  arc A464 (53.3233, 60.5) -> (52.9958, 59.6222) centre (53.3233, 60) ccw
  arc A465 (59.6222, 52.9958) -> (60.5, 53.3233) centre (60, 53.3233) ccw
  line L320 (75.1447, 131.3324) -> (80.089, 122.2131)
  arc A466 (78.848, 118.7118) -> (80.089, 122.2131) centre (77.8913, 121.0215) ccw
  line L321 (64.8827, 112.9272) -> (78.848, 118.7118)
  arc A467 (65.314, 122.1239) -> (72.401, 134.8209) centre (11.7536, 160.3459) ccw
  arc A468 (63.5, 122.7047) -> (65.314, 122.1239) centre (64.5, 122.7047) ccw
  arc A469 (72.401, 134.8209) -> (72.3159, 136.55) centre (70.5576, 135.5967) ccw
  line L322 (63.5, 115.4267) -> (63.5, 113.8511)
  arc A470 (63.5, 113.8511) -> (64.8827, 112.9272) centre (64.5, 113.8511) ccw
  line L323 (49.2953, 108.5) -> (29.964, 108.5)
  arc A471 (40.7299, 98.6445) -> (55.928, 108.2639) centre (13.4685, 158.5315) ccw
  arc A472 (56.5733, 108.5) -> (55.928, 108.2639) centre (56.5733, 107.5) ccw
  arc A473 (40.7299, 98.6445) -> (40.6676, 96.8553) centre (41.1442, 97.7344) ccw
  arc A474 (23.0414, 106.0969) -> (28.9832, 108.2996) centre (3.1615, 168.8384) ccw
  arc A475 (29.964, 108.5) -> (28.9832, 108.2996) centre (29.964, 106) ccw
  arc A476 (23.0414, 106.0969) -> (21.3275, 103.2) centre (23.9793, 103.5865) ccw
  line L324 (33.692, 100.6373) -> (35.45, 99.6841)
  line L325 (25.5, 101) -> (32.2621, 101)
  arc A477 (33.692, 100.6373) -> (32.2621, 101) centre (32.2621, 98) ccw
  line L326 (40.6676, 96.8553) -> (49.7869, 91.911)
  arc A478 (49.7869, 91.911) -> (53.2882, 93.152) centre (50.9785, 94.1087) ccw
  line L327 (59.0728, 107.1173) -> (53.2882, 93.152)
  arc A479 (37.1791, 99.599) -> (49.8761, 106.686) centre (11.6541, 160.2464) ccw
  arc A480 (49.8761, 106.686) -> (49.2953, 108.5) centre (49.2953, 107.5) ccw
  arc A481 (35.45, 99.6841) -> (37.1791, 99.599) centre (36.4033, 101.4424) ccw
  line L328 (56.5733, 108.5) -> (58.1489, 108.5)
  arc A482 (59.0728, 107.1173) -> (58.1489, 108.5) centre (58.1489, 107.5) ccw
  line L329 (122.7047, 63.5) -> (142.036, 63.5)
  arc A483 (131.2701, 73.3555) -> (116.072, 63.7361) centre (158.5315, 13.4685) ccw
  arc A484 (115.4267, 63.5) -> (116.072, 63.7361) centre (115.4267, 64.5) ccw
  arc A485 (131.2701, 73.3555) -> (131.3324, 75.1447) centre (130.8558, 74.2656) ccw
  arc A486 (148.9586, 65.9031) -> (143.0168, 63.7004) centre (168.8384, 3.1616) ccw
  arc A487 (142.036, 63.5) -> (143.0168, 63.7004) centre (142.036, 66) ccw
  arc A488 (148.9586, 65.9031) -> (150.6725, 68.8) centre (148.0207, 68.4135) ccw
  line L330 (138.308, 71.3627) -> (136.55, 72.3159)
  line L331 (146.5, 71) -> (139.7379, 71)
  arc A489 (138.308, 71.3627) -> (139.7379, 71) centre (139.7379, 74) ccw
  line L332 (131.3324, 75.1447) -> (122.2131, 80.089)
  arc A490 (122.2131, 80.089) -> (118.7118, 78.848) centre (121.0215, 77.8913) ccw
  line L333 (112.9272, 64.8827) -> (118.7118, 78.848)
  arc A491 (134.8209, 72.401) -> (122.1239, 65.314) centre (160.3459, 11.7536) ccw
  arc A492 (122.1239, 65.314) -> (122.7047, 63.5) centre (122.7047, 64.5) ccw
  arc A493 (136.55, 72.3159) -> (134.8209, 72.401) centre (135.5967, 70.5576) ccw
  line L334 (115.4267, 63.5) -> (113.8511, 63.5)
  arc A494 (112.9272, 64.8827) -> (113.8511, 63.5) centre (113.8511, 64.5) ccw
  line L335 (108.5, 49.2953) -> (108.5, 29.964)
  arc A495 (108.2639, 55.928) -> (98.6445, 40.7299) centre (158.5315, 13.4685) ccw
  arc A496 (108.2639, 55.928) -> (108.5, 56.5733) centre (107.5, 56.5733) ccw
  arc A497 (96.8553, 40.6676) -> (98.6445, 40.7299) centre (97.7344, 41.1442) ccw
  arc A498 (108.2996, 28.9832) -> (106.0968, 23.0414) centre (168.8384, 3.1616) ccw
  arc A499 (108.2996, 28.9832) -> (108.5, 29.964) centre (106, 29.964) ccw
  arc A500 (103.2, 21.3275) -> (106.0968, 23.0414) centre (103.5865, 23.9793) ccw
  line L336 (100.6373, 33.692) -> (99.6841, 35.45)
  line L337 (101, 25.5) -> (101, 32.2621)
  arc A501 (101, 32.2621) -> (100.6373, 33.692) centre (98, 32.2621) ccw
  line L338 (96.8553, 40.6676) -> (91.911, 49.7869)
  arc A502 (93.152, 53.2882) -> (91.911, 49.7869) centre (94.1087, 50.9785) ccw
  line L339 (107.1173, 59.0728) -> (93.152, 53.2882)
  arc A503 (106.686, 49.8761) -> (99.599, 37.1791) centre (160.2464, 11.6541) ccw
  arc A504 (108.5, 49.2953) -> (106.686, 49.8761) centre (107.5, 49.2953) ccw
  arc A505 (99.599, 37.1791) -> (99.6841, 35.45) centre (101.4423, 36.4033) ccw
  line L340 (108.5, 56.5733) -> (108.5, 58.1489)
  arc A506 (108.5, 58.1489) -> (107.1173, 59.0728) centre (107.5, 58.1489) ccw
  line L341 (63.5, 49.2953) -> (63.5, 29.964)
  arc A507 (73.3555, 40.7299) -> (63.7361, 55.928) centre (13.4685, 13.4685) ccw
  arc A508 (63.5, 56.5733) -> (63.7361, 55.928) centre (64.5, 56.5733) ccw
  arc A509 (73.3555, 40.7299) -> (75.1447, 40.6676) centre (74.2656, 41.1442) ccw
  arc A510 (65.9031, 23.0414) -> (63.7004, 28.9832) centre (3.1615, 3.1616) ccw
  arc A511 (63.5, 29.964) -> (63.7004, 28.9832) centre (66, 29.964) ccw
  arc A512 (65.9031, 23.0414) -> (68.8, 21.3275) centre (68.4135, 23.9793) ccw
  line L342 (71.3627, 33.692) -> (72.3159, 35.45)
  line L343 (71, 25.5) -> (71, 32.2621)
  arc A513 (71.3627, 33.692) -> (71, 32.2621) centre (74, 32.2621) ccw
  line L344 (75.1447, 40.6676) -> (80.089, 49.7869)
  arc A514 (80.089, 49.7869) -> (78.848, 53.2882) centre (77.8913, 50.9785) ccw
  line L345 (64.8827, 59.0728) -> (78.848, 53.2882)
  arc A515 (72.401, 37.1791) -> (65.314, 49.8761) centre (11.7536, 11.6541) ccw
  arc A516 (65.314, 49.8761) -> (63.5, 49.2953) centre (64.5, 49.2953) ccw
  arc A517 (72.3159, 35.45) -> (72.401, 37.1791) centre (70.5576, 36.4033) ccw
  line L346 (63.5, 56.5733) -> (63.5, 58.1489)
  arc A518 (64.8827, 59.0728) -> (63.5, 58.1489) centre (64.5, 58.1489) ccw
  line L347 (49.2953, 63.5) -> (29.964, 63.5)
  arc A519 (55.928, 63.7361) -> (40.7299, 73.3555) centre (13.4685, 13.4685) ccw
  arc A520 (55.928, 63.7361) -> (56.5733, 63.5) centre (56.5733, 64.5) ccw
  arc A521 (40.6676, 75.1447) -> (40.7299, 73.3555) centre (41.1442, 74.2656) ccw
  arc A522 (28.9832, 63.7004) -> (23.0414, 65.9031) centre (3.1615, 3.1616) ccw
  arc A523 (28.9832, 63.7004) -> (29.964, 63.5) centre (29.964, 66) ccw
  arc A524 (21.3275, 68.8) -> (23.0414, 65.9031) centre (23.9793, 68.4135) ccw
  line L348 (33.692, 71.3627) -> (35.45, 72.3159)
  line L349 (25.5, 71) -> (32.2621, 71)
  arc A525 (32.2621, 71) -> (33.692, 71.3627) centre (32.2621, 74) ccw
  line L350 (40.6676, 75.1447) -> (49.7869, 80.089)
  arc A526 (53.2882, 78.848) -> (49.7869, 80.089) centre (50.9785, 77.8913) ccw
  line L351 (59.0728, 64.8827) -> (53.2882, 78.848)
  arc A527 (49.8761, 65.314) -> (37.1791, 72.401) centre (11.6541, 11.7536) ccw
  arc A528 (49.2953, 63.5) -> (49.8761, 65.314) centre (49.2953, 64.5) ccw
  arc A529 (37.1791, 72.401) -> (35.45, 72.3159) centre (36.4033, 70.5576) ccw
  line L352 (56.5733, 63.5) -> (58.1489, 63.5)
  arc A530 (58.1489, 63.5) -> (59.0728, 64.8827) centre (58.1489, 64.5) ccw
  line L353 (108.5, 122.7047) -> (108.5, 142.036)
  arc A531 (98.6445, 131.2701) -> (108.2639, 116.072) centre (158.5315, 158.5315) ccw
  arc A532 (108.5, 115.4267) -> (108.2639, 116.072) centre (107.5, 115.4267) ccw
  arc A533 (98.6445, 131.2701) -> (96.8553, 131.3324) centre (97.7344, 130.8558) ccw
  arc A534 (106.0968, 148.9586) -> (108.2996, 143.0168) centre (168.8384, 168.8384) ccw
  arc A535 (108.5, 142.036) -> (108.2996, 143.0168) centre (106, 142.036) ccw
  arc A536 (106.0968, 148.9586) -> (103.2, 150.6725) centre (103.5865, 148.0207) ccw
  line L354 (100.6373, 138.308) -> (99.6841, 136.55)
  line L355 (101, 146.5) -> (101, 139.7379)
  arc A537 (100.6373, 138.308) -> (101, 139.7379) centre (98, 139.7379) ccw
  line L356 (96.8553, 131.3324) -> (91.911, 122.2131)
  arc A538 (91.911, 122.2131) -> (93.152, 118.7118) centre (94.1087, 121.0215) ccw
  line L357 (107.1173, 112.9272) -> (93.152, 118.7118)
  arc A539 (99.599, 134.8209) -> (106.686, 122.1239) centre (160.2464, 160.3459) ccw
  arc A540 (106.686, 122.1239) -> (108.5, 122.7047) centre (107.5, 122.7047) ccw
  arc A541 (99.6841, 136.55) -> (99.599, 134.8209) centre (101.4423, 135.5967) ccw
  line L358 (108.5, 115.4267) -> (108.5, 113.8511)
  arc A542 (107.1173, 112.9272) -> (108.5, 113.8511) centre (107.5, 113.8511) ccw
  line L359 (122.7047, 108.5) -> (142.036, 108.5)
  arc A543 (116.072, 108.2639) -> (131.2701, 98.6445) centre (158.5315, 158.5315) ccw
  arc A544 (116.072, 108.2639) -> (115.4267, 108.5) centre (115.4267, 107.5) ccw
  arc A545 (131.3324, 96.8553) -> (131.2701, 98.6445) centre (130.8558, 97.7344) ccw
  arc A546 (143.0168, 108.2996) -> (148.9586, 106.0969) centre (168.8384, 168.8384) ccw
  arc A547 (143.0168, 108.2996) -> (142.036, 108.5) centre (142.036, 106) ccw
  arc A548 (150.6725, 103.2) -> (148.9586, 106.0969) centre (148.0207, 103.5865) ccw
  line L360 (138.308, 100.6373) -> (136.55, 99.6841)
  line L361 (146.5, 101) -> (139.7379, 101)
  arc A549 (139.7379, 101) -> (138.308, 100.6373) centre (139.7379, 98) ccw
  line L362 (131.3324, 96.8553) -> (122.2131, 91.911)
  arc A550 (118.7118, 93.152) -> (122.2131, 91.911) centre (121.0215, 94.1087) ccw
  line L363 (112.9272, 107.1173) -> (118.7118, 93.152)
  arc A551 (122.1239, 106.686) -> (134.8209, 99.599) centre (160.3459, 160.2464) ccw
  arc A552 (122.7047, 108.5) -> (122.1239, 106.686) centre (122.7047, 107.5) ccw
  arc A553 (134.8209, 99.599) -> (136.55, 99.6841) centre (135.5967, 101.4424) ccw
  line L364 (115.4267, 108.5) -> (113.8511, 108.5)
  arc A554 (113.8511, 108.5) -> (112.9272, 107.1173) centre (113.8511, 107.5) ccw
  line L365 (21.3275, 103.2) -> (25.5, 103.2)
  line L366 (25.5, 103.2) -> (25.5, 101)
  line L367 (21.3275, 68.8) -> (25.5, 68.8)
  line L368 (25.5, 68.8) -> (25.5, 71)
  line L369 (150.6725, 103.2) -> (146.5, 103.2)
  line L370 (146.5, 103.2) -> (146.5, 101)
  line L371 (150.6725, 68.8) -> (146.5, 68.8)
  line L372 (146.5, 68.8) -> (146.5, 71)
  line L373 (68.8, 150.6725) -> (68.8, 146.5)
  line L374 (68.8, 146.5) -> (71, 146.5)
  line L375 (103.2, 150.6725) -> (103.2, 146.5)
  line L376 (103.2, 146.5) -> (101, 146.5)
  line L377 (68.8, 21.3275) -> (68.8, 25.5)
  line L378 (68.8, 25.5) -> (71, 25.5)
  line L379 (103.2, 21.3275) -> (103.2, 25.5)
  line L380 (103.2, 25.5) -> (101, 25.5)
  point P0 (0, 0)
  constraints: 504 point on circle, 382 end point, 278 centre point, 225 tangent, 125 horizontal, 125 vertical, 24 perpendicular, 21 coincident, 7 collinear, 7 parallel, 1 point on line, 628 other
extrude "Extrusion2" add sketch "Sketch1" along normal blind 2 contours L0 L1 L2 L3 L4 A27 L11 A28 A30 A29 A31 A32 L5 A34 L12 A33 L6 L7 L8 L9 L10 A47 L18 L19 L20 L21 L22 A55 L30 A54 A53 A52 A51 L23 A49 L29 A50 A48 L28 L27 L26 L25 L24 A46 L31 L32 L33 L34 L35 A62 L43 A61 A60 A59 A58 L36 A57 L42 A56 L41 L40 L39 L38 L37 A45 L44 L45 L46 L47 L48 A69 L56 A68 A67 A66 A65 L54 A64 L55 A63 L53 L52 L51 L50 L49 A44
sketch "Sketch2" plane through (0, 2, 0) normal (0, 1, 0) x (1, 0, 0)
  line L0 (-55.8078, -89.9295) -> (-61.8724, -104.5705) projected
  line L1 (-67.4295, -110.1276) -> (-82.0705, -116.1922) projected
  line L2 (-89.9295, -116.1922) -> (-104.5705, -110.1276) projected
  line L3 (-110.1276, -104.5705) -> (-116.1922, -89.9295) projected
  line L4 (-116.1922, -82.0705) -> (-110.1276, -67.4295) projected
  line L5 (-104.5705, -61.8724) -> (-89.9295, -55.8078) projected
  line L6 (-82.0705, -55.8078) -> (-67.4295, -61.8724) projected
  line L7 (-61.8724, -67.4295) -> (-55.8078, -82.0705) projected
  line L8 (-97.25, -113.1599) -> (-74.75, -58.8401)
  line L9 (-74.75, -113.1599) -> (-97.25, -58.8401)
  line L10 (-113.1599, -74.75) -> (-58.8401, -97.25)
  line L11 (-58.8401, -74.75) -> (-113.1599, -97.25)
  line L12 (-97.25, -113.1599) -> (-96.3261, -113.5426)
  line L13 (-96.3261, -113.5426) -> (-73.8261, -59.2228)
  line L14 (-73.8261, -59.2228) -> (-75.6739, -58.4574)
  line L15 (-75.6739, -58.4574) -> (-98.1739, -112.7772)
  line L16 (-97.25, -113.1599) -> (-98.1739, -112.7772)
  line L17 (-74.75, -113.1599) -> (-73.8261, -112.7772)
  line L18 (-73.8261, -112.7772) -> (-96.3261, -58.4574)
  line L19 (-96.3261, -58.4574) -> (-98.1739, -59.2228)
  line L20 (-98.1739, -59.2228) -> (-75.6739, -113.5426)
  line L21 (-74.75, -113.1599) -> (-75.6739, -113.5426)
  line L22 (-58.8401, -97.25) -> (-58.4574, -96.3261)
  line L23 (-58.4574, -96.3261) -> (-112.7772, -73.8261)
  line L24 (-112.7772, -73.8261) -> (-113.5426, -75.6739)
  line L25 (-113.5426, -75.6739) -> (-59.2228, -98.1739)
  line L26 (-59.2228, -98.1739) -> (-58.8401, -97.25)
  line L27 (-58.8401, -74.75) -> (-58.4574, -75.6739)
  line L28 (-58.4574, -75.6739) -> (-112.7772, -98.1739)
  line L29 (-112.7772, -98.1739) -> (-113.5426, -96.3261)
  line L30 (-113.5426, -96.3261) -> (-59.2228, -73.8261)
  line L31 (-58.8401, -74.75) -> (-59.2228, -73.8261)
  dimension "d4" = 1
  dimension "d5" = 2
  dimension "d6" = 1
  dimension "d7" = 2
  dimension "d8" = 1
  dimension "d9" = 2
  dimension "d10" = 1
  dimension "d11" = 2
  constraints: 48 end point, 16 point on line, 10 perpendicular, 8 midpoint, 2 collinear
  measures "d4" distance of L8.start L12.end
  measures "d5" distance of L13.end L14.end
  measures "d6" distance of L9.start L17.end
  measures "d7" distance of L18.end L19.end
  measures "d8" distance of L10.end L22.end
  measures "d9" distance of L23.end L24.end
  measures "d10" distance of L11.start L27.end
  measures "d11" distance of L28.end L29.end
extrude "Extrusion3" add sketch "Sketch2" against normal blind 2
fillet "Fillet1" radius 2 16 edges at (-112.7772, 1, 98.1739) (-113.5426, 1, 96.3261) (-98.1739, 1, 112.7772) (-96.3261, 1, 113.5426) (-112.7772, 1, 73.8261) (-113.5426, 1, 75.6739) (-98.1739, 1, 59.2228) (-96.3261, 1, 58.4574) (-73.8261, 1, 59.2228) (-75.6739, 1, 58.4574) (-58.4574, 1, 75.6739) (-59.2228, 1, 73.8261) (-59.2228, 1, 98.1739) (-58.4574, 1, 96.3261) (-75.6739, 1, 113.5426) (-73.8261, 1, 112.7772)
fillet "Fillet1" radius 2 8 edges at (-87.8478, 1, 87.8478) (-86, 1, 88.6131) (-84.1522, 1, 87.8478) (-83.3869, 1, 86) (-84.1522, 1, 84.1522) (-86, 1, 83.3869) (-87.8478, 1, 84.1522) (-88.6131, 1, 86)
sketch "Sketch3" plane through (0, 2, 0) normal (0, 1, 0) x (1, 0, 0)
  circle A0 centre (-86, -86) radius 1.6002
  dimension "d16" = 3.2004
  constraints: 1 centre point
  measures "d16" diameter of A0
extrude "Extrusion4" cut sketch "Sketch3" against normal blind 2
body "Solid2"
